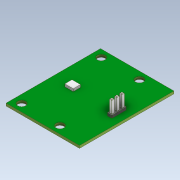
# Autodesk Inventor part: LED8
Saved by Autodesk Inventor 2020 (Build 240168000, 168)
## iProperties
Created: 2020-09-03
Part Number: LED8
Material: Generic
Document SubType Name: Modeling
Designer: Admin
Density: 1 g/cm^3
Appearance: Olive Green
Author: Admin
Autodesk Inventor part; units mm, degrees
ref_plane "YZ Plane" through (0, 0, 0) normal (1, 0, 0) x (0, 1, 0)
ref_plane "XZ Plane" through (0, 0, 0) normal (0, 1, 0) x (-1, 0, 0)
ref_plane "XY Plane" through (0, 0, 0) normal (0, 0, 1) x (1, 0, 0)
sketch "Sketch1" plane through (0, 0, 0) normal (0, 1, 0) x (-1, 0, 0)
  line L0 (0, 0) -> (30, 0)
  line L1 (30, 0) -> (30, -38.6)
  line L2 (30, -38.6) -> (0, -38.6)
  line L3 (0, -38.6) -> (0, 0)
  dimension "d0" = 30
  dimension "d1" = 38.6
  constraints: 8 end point, 2 parallel, 1 horizontal, 1 perpendicular
  measures "d0" distance of L0.start L0.end
  measures "d1" distance of L0.end L1.end
extrude "Extrusion1" add sketch "Sketch1" along normal blind 1
sketch "Sketch2" plane through (0, 1, 0) normal (0, 1, 0) x (1, 0, 0)
  line L0 (-23.842, 17.8) -> (-20.342, 17.8)
  line L1 (-20.342, 17.8) -> (-20.342, 20.8)
  line L2 (-20.342, 20.8) -> (-23.842, 20.8)
  line L3 (-23.842, 20.8) -> (-23.842, 17.8)
  line L4 (-30, 0) -> (0, 0) projected
  line L5 (-30, 38.6) -> (-30, 0) projected
  dimension "d4" = 3
  dimension "d5" = 3.5
  dimension "d6" = 17.8
  dimension "d7" = 6.158
  constraints: 8 end point, 2 parallel, 1 horizontal, 1 perpendicular
  measures "d4" distance of L2.end L0.start
  measures "d5" distance of L1.end L2.end
  measures "d6" distance between parallel lines of L0 L4
  measures "d7" distance between parallel lines of L5 L3
extrude "Extrusion2" add sketch "Sketch2" along normal blind 1
sketch "Sketch3" plane through (0, 1, 0) normal (0, 1, 0) x (1, 0, 0)
  line L0 (-5, 16.26) -> (-3, 16.26)
  line L1 (-3, 16.26) -> (-3, 22.34)
  line L2 (-3, 22.34) -> (-5, 22.34)
  line L3 (-5, 22.34) -> (-5, 16.26)
  line L4 (-30, 0) -> (0, 0) projected
  line L5 (0, 0) -> (0, 38.6) projected
  dimension "d10" = 2
  dimension "d11" = 6.08
  dimension "d12" = 16.26
  dimension "d13" = 3
  constraints: 8 end point, 2 parallel, 1 horizontal, 1 perpendicular
  measures "d10" distance of L1.end L2.end
  measures "d11" distance of L2.end L0.start
  measures "d12" distance between parallel lines of L0 L4
  measures "d13" distance between parallel lines of L5 L1
extrude "Extrusion3" add sketch "Sketch3" along normal blind 1
chamfer "Chamfer1" distance 0.2 angle 45 4 edges at (-5, 1.5, -16.26) (-3, 1.5, -16.26) (-5, 1.5, -22.34) (-3, 1.5, -22.34)
sketch "Sketch5" plane through (0, 2, 0) normal (0, 1, 0) x (1, 0, 0)
  line L0 (-4.5, 16.76) -> (-3.5, 16.76)
  line L1 (-3.5, 16.76) -> (-3.5, 17.76)
  line L2 (-3.5, 17.76) -> (-4.5, 17.76)
  line L3 (-4.5, 17.76) -> (-4.5, 16.76)
  line L4 (-4.8, 16.26) -> (-3.2, 16.26) projected
  line L5 (-3, 16.46) -> (-3, 22.14) projected
  point P0 (0, 0)
  dimension "d23" = 1
  dimension "d24" = 1
  dimension "d25" = 0.5
  dimension "d26" = 0.5
  constraints: 8 end point, 2 parallel, 1 horizontal, 1 perpendicular
  measures "d23" distance of L2.end L0.start
  measures "d24" distance of L0.start L0.end
  measures "d25" distance between parallel lines of L4 L0
  measures "d26" distance between parallel lines of L5 L1
extrude "Extrusion4" add sketch "Sketch5" along normal blind 5
pattern_linear "Rectangular Pattern1" count 3 spacing 2.04 along (0, 0, -1) of "Extrusion4"
chamfer "Chamfer2" distance 0.2 angle 45 12 edges at (-4.5, 7, -17.26) (-4, 7, -17.76) (-4, 7, -16.76) (-3.5, 7, -17.26) (-4, 7, -18.8) (-4.5, 7, -19.3) (-4, 7, -19.8) (-3.5, 7, -19.3) (-4, 7, -20.84) (-4.5, 7, -21.34) (-4, 7, -21.84) (-3.5, 7, -21.34)
sketch "Sketch6" plane through (0, 1, 0) normal (0, 1, 0) x (1, 0, 0)
  circle A0 centre (-26.676, 3.059) radius 1.6
  circle A1 centre (-11.026, 3.059) radius 1.6
  circle A2 centre (-11.026, 35.541) radius 1.6
  circle A3 centre (-26.676, 35.541) radius 1.6
  line L0 (0, 38.6) -> (-30, 38.6) projected
  line L1 (-30, 38.6) -> (-30, 0) projected
  point P0 (0, 0)
  dimension "d35" = 3.2
  dimension "d36" = 3.2
  dimension "d37" = 3.2
  dimension "d38" = 3.2
  dimension "d39" = 15.65
  dimension "d40" = 15.65
  dimension "d41" = 32.482
  dimension "d42" = 0
  dimension "d43" = 0
  dimension "d44" = 0
  dimension "d45" = 3.059
  dimension "d46" = 3.324
  constraints: 4 centre point
  measures "d35" diameter of A0
  measures "d36" diameter of A1
  measures "d37" diameter of A2
  measures "d38" diameter of A3
  measures "d39" distance of A0.centre A1.centre
  measures "d40" distance of A3.centre A2.centre
  measures "d41" distance of A2.centre A1.centre
  measures "d42" horizontal distance of A2.centre A1.centre
  measures "d43" vertical distance of A1.centre A0.centre
  measures "d44" vertical distance of A2.centre A3.centre
  measures "d45" distance from line of L0 A2.centre
  measures "d46" distance from line of L1 A0.centre
extrude "Extrusion5" cut sketch "Sketch6" against normal blind 5
body "Solid1"
